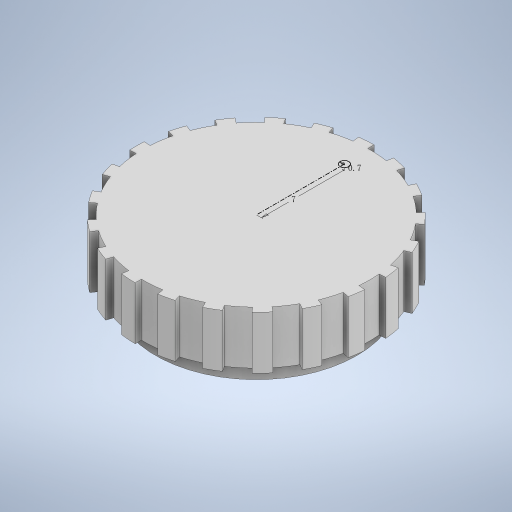
# Autodesk Inventor part: rot_no_val_th
Saved by Autodesk Inventor 2023 (Build 270158000, 158)
## iProperties
Created: 2023-05-20
Part Number: rot_no_val_th
Material: 常规
Document SubType Name: Modeling
Designer: LiuZeshu
Density: 1 g/cm^3
Appearance: 默认
Author: LiuZeshu
Autodesk Inventor part; units mm, degrees
ref_plane "YZ Plane" through (0, 0, 0) normal (1, 0, 0) x (0, 1, 0)
ref_plane "XZ Plane" through (0, 0, 0) normal (0, 1, 0) x (-1, 0, 0)
ref_plane "XY Plane" through (0, 0, 0) normal (0, 0, 1) x (1, 0, 0)
sketch "草图1" plane through (0, 0, 0) normal (0, 1, 0) x (-1, 0, 0)
  arc A0 (1.5199, -0.5) -> (-1.5199, -0.5) centre (0, 0) ccw
  line L0 (1.5199, -0.5) -> (-1.5199, -0.5)
  circle A1 centre (0, 0) radius 9
  dimension "d0" = 3.2
  dimension "d1" = 2.1
  dimension "d2" = 18
  constraints: 2 centre point, 2 coincident, 2 end point, 2 point on circle, 1 horizontal
  measures "d0" diameter of A0
  measures "d2" diameter of A1
extrude "拉伸1" add sketch "草图1" along normal blind 2.3
sketch "草图2" plane through (0, 2.3, 0) normal (0, 1, 0) x (1, 0, 0)
  circle A0 centre (0, 0) radius 9
  line L0 (-1.5199, 0.5) -> (1.5199, 0.5) projected
  arc A1 (-1.5199, 0.5) -> (1.5199, 0.5) centre (0, 0) ccw
  line L1 (-1.5199, 0.5) -> (1.5199, 0.5)
  circle A2 centre (0, 0) radius 9 projected
  constraints: 2 centre point, 2 coincident, 2 end point, 2 point on circle, 1 collinear, 1 concentric
extrude "拉伸2" add sketch "草图2" along normal blind 0.4 contours A0 | L0 A1
sketch "草图5" plane through (0, 2.7, 0) normal (0, 1, 0) x (1, 0, 0)
  circle A0 centre (0, 7) radius 0.35
  line L0 (0, 7) -> (0, 0)
  dimension "d27" = 0.7
  dimension "d28" = 7
  constraints: 2 end point, 1 centre point, 1 vertical
  measures "d27" diameter of A0
  measures "d28" distance of L0.end L0.start
sketch "草图9" plane through (0, 0, 0) normal (0, -1, 0) x (1, 0, 0)
  circle A0 centre (0, 0) radius 9
  circle A1 centre (0, 0) radius 7
  circle A2 centre (0, 0) radius 9 projected
  dimension "d39" = 14
  constraints: 2 centre point, 2 coincident, 1 concentric
  measures "d39" diameter of A1
extrude "拉伸7" add sketch "草图9" along normal blind 3
sketch "草图6" plane through (0, 2.7, 0) normal (0, 1, 0) x (1, 0, 0)
  arc A0 (-8.9832, 0.5494) -> (-8.9832, -0.5494) centre (0, 0) ccw
  circle A1 centre (0, 0) radius 9 projected
  arc A2 (-1.5199, 0.5) -> (1.5199, 0.5) centre (0, 0) ccw projected
  arc A3 (-9.4823, 0.58) -> (-9.4823, -0.58) centre (0, 0) ccw
  line L0 (-9.4823, -0.58) -> (-8.9832, -0.5494)
  line L1 (-9.4823, 0.58) -> (-8.9832, 0.5494)
  line L2 (-11.1138, 0) -> (0, 0)
  line L3 (-1.5199, 0.5) -> (1.5199, 0.5) projected
  arc A4 (-8.7461, -2.1228) -> (-8.4222, -3.1729) centre (0, 0) ccw
  arc A5 (-9.232, -2.2408) -> (-8.8901, -3.3491) centre (0, 0) ccw
  line L4 (-8.8901, -3.3491) -> (-8.4222, -3.1729)
  line L5 (-9.232, -2.2408) -> (-8.7461, -2.1228)
  line L6 (-10.62, -3.2758) -> (0, 0)
  arc A6 (-7.7318, -4.6065) -> (-7.1128, -5.5144) centre (0, 0) ccw
  arc A7 (-8.1613, -4.8624) -> (-7.5079, -5.8207) centre (0, 0) ccw
  line L7 (-7.5079, -5.8207) -> (-7.1128, -5.5144)
  line L8 (-8.1613, -4.8624) -> (-7.7318, -4.6065)
  line L9 (-9.1826, -6.2606) -> (0, 0)
  arc A8 (-6.0305, -6.6808) -> (-5.1714, -7.3659) centre (0, 0) ccw
  arc A9 (-6.3655, -7.0519) -> (-5.4587, -7.7751) centre (0, 0) ccw
  line L10 (-5.4587, -7.7751) -> (-5.1714, -7.3659)
  line L11 (-6.3655, -7.0519) -> (-6.0305, -6.6808)
  line L12 (-6.9293, -8.6891) -> (0, 0)
  arc A10 (-3.7934, -8.1615) -> (-2.7705, -8.563) centre (0, 0) ccw
  arc A11 (-4.0041, -8.6149) -> (-2.9244, -9.0387) centre (0, 0) ccw
  line L13 (-2.9244, -9.0387) -> (-2.7705, -8.563)
  line L14 (-4.0041, -8.6149) -> (-3.7934, -8.1615)
  line L15 (-4.0603, -10.3455) -> (0, 0)
  arc A12 (-1.2192, -8.917) -> (-0.1234, -8.9992) centre (0, 0) ccw
  arc A13 (-1.287, -9.4124) -> (-0.1303, -9.4991) centre (0, 0) ccw
  line L16 (-0.1303, -9.4991) -> (-0.1234, -8.9992)
  line L17 (-1.287, -9.4124) -> (-1.2192, -8.917)
  line L18 (-0.8305, -11.0827) -> (0, 0)
  arc A14 (1.4633, -8.8802) -> (2.5346, -8.6357) centre (0, 0) ccw
  arc A15 (1.5446, -9.3736) -> (2.6754, -9.1155) centre (0, 0) ccw
  line L19 (2.6754, -9.1155) -> (2.5346, -8.6357)
  line L20 (1.5446, -9.3736) -> (1.4633, -8.8802)
  line L21 (2.4731, -10.8351) -> (0, 0)
  arc A16 (4.0158, -8.0544) -> (4.9674, -7.505) centre (0, 0) ccw
  arc A17 (4.2389, -8.5019) -> (5.2434, -7.9219) centre (0, 0) ccw
  line L22 (5.2434, -7.9219) -> (4.9674, -7.505)
  line L23 (4.2389, -8.5019) -> (4.0158, -8.0544)
  line L24 (5.5569, -9.6248) -> (0, 0)
  arc A18 (6.2114, -6.5129) -> (6.9589, -5.7074) centre (0, 0) ccw
  arc A19 (6.5565, -6.8747) -> (7.3455, -6.0244) centre (0, 0) ccw
  line L25 (7.3455, -6.0244) -> (6.9589, -5.7074)
  line L26 (6.5565, -6.8747) -> (6.2114, -6.5129)
  line L27 (8.147, -7.5593) -> (0, 0)
  arc A20 (7.8552, -4.3927) -> (8.332, -3.4026) centre (0, 0) ccw
  arc A21 (8.2916, -4.6367) -> (8.7949, -3.5917) centre (0, 0) ccw
  line L28 (8.7949, -3.5917) -> (8.332, -3.4026)
  line L29 (8.2916, -4.6367) -> (7.8552, -4.3927)
  line L30 (10.0132, -4.8221) -> (0, 0)
  arc A22 (8.801, -1.8822) -> (8.9648, -0.7956) centre (0, 0) ccw
  arc A23 (9.2899, -1.9867) -> (9.4628, -0.8398) centre (0, 0) ccw
  line L31 (9.4628, -0.8398) -> (8.9648, -0.7956)
  line L32 (9.2899, -1.9867) -> (8.801, -1.8822)
  line L33 (10.9897, -1.6564) -> (0, 0)
  arc A24 (8.9648, 0.7956) -> (8.801, 1.8822) centre (0, 0) ccw
  arc A25 (9.4628, 0.8398) -> (9.2899, 1.9867) centre (0, 0) ccw
  line L34 (9.2899, 1.9867) -> (8.801, 1.8822)
  line L35 (9.4628, 0.8398) -> (8.9648, 0.7956)
  line L36 (10.9897, 1.6564) -> (0, 0)
  arc A26 (8.332, 3.4026) -> (7.8552, 4.3927) centre (0, 0) ccw
  arc A27 (8.7949, 3.5917) -> (8.2916, 4.6367) centre (0, 0) ccw
  line L37 (8.2916, 4.6367) -> (7.8552, 4.3927)
  line L38 (8.7949, 3.5917) -> (8.332, 3.4026)
  line L39 (10.0132, 4.8221) -> (0, 0)
  arc A28 (6.9589, 5.7074) -> (6.2114, 6.5129) centre (0, 0) ccw
  arc A29 (7.3455, 6.0244) -> (6.5565, 6.8747) centre (0, 0) ccw
  line L40 (6.5565, 6.8747) -> (6.2114, 6.5129)
  line L41 (7.3455, 6.0244) -> (6.9589, 5.7074)
  line L42 (8.147, 7.5593) -> (0, 0)
  arc A30 (4.9674, 7.505) -> (4.0158, 8.0544) centre (0, 0) ccw
  arc A31 (5.2434, 7.9219) -> (4.2389, 8.5019) centre (0, 0) ccw
  line L43 (4.2389, 8.5019) -> (4.0158, 8.0544)
  line L44 (5.2434, 7.9219) -> (4.9674, 7.505)
  line L45 (5.5569, 9.6248) -> (0, 0)
  arc A32 (2.5346, 8.6357) -> (1.4633, 8.8802) centre (0, 0) ccw
  arc A33 (2.6754, 9.1155) -> (1.5446, 9.3736) centre (0, 0) ccw
  line L46 (1.5446, 9.3736) -> (1.4633, 8.8802)
  line L47 (2.6754, 9.1155) -> (2.5346, 8.6357)
  line L48 (2.4731, 10.8351) -> (0, 0)
  arc A34 (-0.1234, 8.9992) -> (-1.2192, 8.917) centre (0, 0) ccw
  arc A35 (-0.1303, 9.4991) -> (-1.287, 9.4124) centre (0, 0) ccw
  line L49 (-1.287, 9.4124) -> (-1.2192, 8.917)
  line L50 (-0.1303, 9.4991) -> (-0.1234, 8.9992)
  line L51 (-0.8305, 11.0827) -> (0, 0)
  arc A36 (-2.7705, 8.563) -> (-3.7934, 8.1615) centre (0, 0) ccw
  arc A37 (-2.9244, 9.0387) -> (-4.0041, 8.6149) centre (0, 0) ccw
  line L52 (-4.0041, 8.6149) -> (-3.7934, 8.1615)
  line L53 (-2.9244, 9.0387) -> (-2.7705, 8.563)
  line L54 (-4.0603, 10.3455) -> (0, 0)
  arc A38 (-5.1714, 7.3659) -> (-6.0305, 6.6808) centre (0, 0) ccw
  arc A39 (-5.4587, 7.7751) -> (-6.3655, 7.0519) centre (0, 0) ccw
  line L55 (-6.3655, 7.0519) -> (-6.0305, 6.6808)
  line L56 (-5.4587, 7.7751) -> (-5.1714, 7.3659)
  line L57 (-6.9293, 8.6891) -> (0, 0)
  arc A40 (-7.1128, 5.5144) -> (-7.7318, 4.6065) centre (0, 0) ccw
  arc A41 (-7.5079, 5.8207) -> (-8.1613, 4.8624) centre (0, 0) ccw
  line L58 (-8.1613, 4.8624) -> (-7.7318, 4.6065)
  line L59 (-7.5079, 5.8207) -> (-7.1128, 5.5144)
  line L60 (-9.1826, 6.2606) -> (0, 0)
  arc A42 (-8.4222, 3.1729) -> (-8.7461, 2.1228) centre (0, 0) ccw
  arc A43 (-8.8901, 3.3491) -> (-9.232, 2.2408) centre (0, 0) ccw
  line L61 (-9.232, 2.2408) -> (-8.7461, 2.1228)
  line L62 (-8.8901, 3.3491) -> (-8.4222, 3.1729)
  line L63 (-10.62, 3.2758) -> (0, 0)
  point P0 (7.8552, 4.3927)
  point P1 (8.332, 3.4026)
  point P2 (6.2114, 6.5129)
  point P3 (6.9589, 5.7074)
  point P4 (4.9674, 7.505)
  point P5 (1.4633, 8.8802)
  point P6 (2.5346, 8.6357)
  point P7 (-1.2192, 8.917)
  point P8 (-0.1234, 8.9992)
  point P9 (-3.7934, 8.1615)
  point P10 (-2.7705, 8.563)
  point P11 (-5.1714, 7.3659)
  point P12 (-7.7318, 4.6065)
  point P13 (-7.1128, 5.5144)
  point P14 (-8.7461, 2.1228)
  point P15 (-7.1128, -5.5144)
  point P16 (-7.7318, -4.6065)
  point P17 (-5.1714, -7.3659)
  point P18 (-6.0305, -6.6808)
  point P19 (-3.7934, -8.1615)
  point P20 (-0.1234, -8.9992)
  point P21 (-1.2192, -8.917)
  point P22 (2.5346, -8.6357)
  point P23 (1.4633, -8.8802)
  point P24 (4.9674, -7.505)
  point P25 (4.0158, -8.0544)
  point P26 (6.9589, -5.7074)
  point P27 (6.2114, -6.5129)
  point P28 (8.332, -3.4026)
  point P29 (7.8552, -4.3927)
  point P30 (8.9648, -0.7956)
  point P31 (8.801, -1.8822)
  point P32 (8.801, 1.8822)
  point P33 (8.9648, 0.7956)
  dimension "d31" = 0.5
  dimension "d32" = 7
  dimension "d35" = 360
  constraints: 126 end point, 84 point on circle, 44 coincident, 42 centre point, 42 point on line, 1 parallel, 298 other
  measures "d31" radial gap between concentric circles of A3 A0
  measures "d32" angle of L1 L0
extrude "拉伸6" add sketch "草图6" against normal up to surface (5.7 mm away) contours A0 L2 A3 L1 | A0 L0 A3 L2 | L61 A43 L63 A1 | L63 A43 L62 A1 | A1 L6 A5 L5 | A1 L4 A5 L6 | L58 A41 L60 A1 | L9 A7 L8 A1 | A1 L7 A7 L9 | L12 A9 L11 A1 | A1 L10 A9 L12 | L15 A11 L14 A1 | A1 L13 A11 L15 | L18 A13 L17 A1 | A1 L16 A13 L18 | L21 A15 L20 A1 | A1 L19 A15 L21 | L24 A17 L23 A1 | A1 L22 A17 L24 | L27 A19 L26 A1 | A1 L25 A19 L27 | L30 A21 L29 A1 | A1 L28 A21 L30 | L33 A23 L32 A1 | A1 L31 A23 L33 | L36 A25 L35 A1 | A1 L34 A25 L36 | L39 A27 L38 A1 | A1 L37 A27 L39 | L42 A29 L41 A1 | A1 L40 A29 L42 | L45 A31 L44 A1 | A1 L43 A31 L45 | L48 A33 L47 A1 | A1 L46 A33 L48 | L51 A35 L50 A1 | A1 L49 A35 L51 | L54 A37 L53 A1 | A1 L52 A37 L54 | L57 A39 L56 A1 | A1 L55 A39 L57 | L60 A41 L59 A1
sketch "草图7" plane through (0, 0, 0) normal (0, -1, 0) x (1, 0, 0)
  point P0 (0, 0)
sketch "草图8" plane through (0, 0, 0) normal (0, -1, 0) x (1, 0, 0)
  point P0 (0, 0)
sketch "草图10" plane through (0, -3, 0) normal (0, -1, 0) x (1, 0, 0)
  circle A0 centre (0, 0) radius 8
  circle A1 centre (0, 0) radius 7 projected
  line L0 (8.801, 1.8822) -> (9.2899, 1.9867) projected
  circle A2 centre (0, 0) radius 9.5
  dimension "d42" = 1
  constraints: 2 coincident, 1 centre point, 3 other
  measures "d42" radial gap between concentric circles of A1 A0
extrude "拉伸8" cut sketch "草图10" against normal blind 1.5 contours A2
